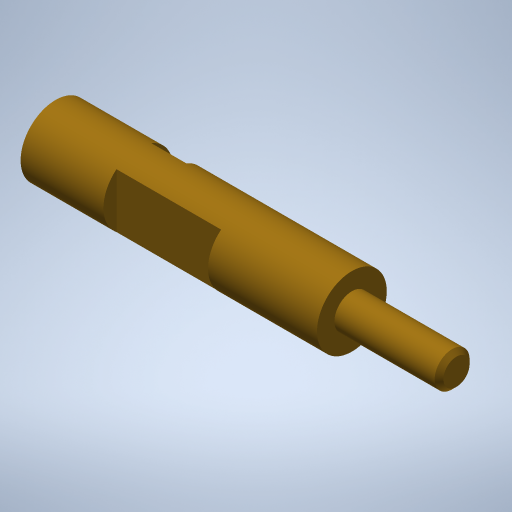
# Autodesk Inventor part: Kurbelwelle
Saved by Autodesk Inventor 2024 (Build 280153000, 153)
## iProperties
Created: 2004-03-27
Part Number: Kurbelwelle
Material: CuZn40
Description: Kurbelwelle
Document SubType Name: Modellieren
Designer: UR
Density: 8.47 g/cm^3
Appearance: Metall - Messing
Control State: 0
Master: False
Checked Out: False
Shininess: 20.0
Angle Display Precision: 2
Document Length Units: 11269
Document Angle Units: 11279
Document Time Units: 11290
Document Mass Units: 11283
Document Length Units Precision: 3
Document Angle Units Precision: 2
Density: 0.0
Volumn: 0.0
Area: 0.0
PropertySet Name: Model Information
Author: UR
Autodesk Inventor part; units mm, degrees
note: some values were not read from the file. Chosen so that the rebuilt part matches the saved one: direction of "3,2 Bohrung radial".
ref_plane "YZ Ebene" through (0, 0, 0) normal (1, 0, 0) x (0, 1, 0)
sketch "Skizze1" plane through (0, 0, 0) normal (0, 0, 1) x (1, 0, 0)
  line L0 (-16.1705, 4.6008) -> (-16.1705, 8.6008)
  line L1 (-16.1705, 8.6008) -> (17.8295, 8.6008)
  line L2 (17.8295, 8.6008) -> (17.8295, 6.6008)
  line L3 (17.8295, 6.6008) -> (29.8295, 6.6008)
  line L4 (29.8295, 6.6008) -> (29.8295, 4.6008)
  line L5 (29.8295, 4.6008) -> (-16.1705, 4.6008)
  dimension "d0" = 46
  dimension "d1" = 12
  dimension "d2" = 4
  dimension "d3" = 8
  constraints: 12 end point, 4 parallel, 1 perpendicular, 1 vertical
  measures "d0" distance of L4.end L0.start
  measures "d1" distance of L2.end L3.end
  measures "d2" diameter of L3 L5
  measures "d3" diameter of L1 L5
revolve "Grundkörper" add sketch "Skizze1" angle 360 about axis through (29.8295, 4.6008, 0) along (-1, 0, 0)
sketch "Skizze2" plane through (-16.1705, 4.6008, 0) normal (-1, 0, 0) x (0, 0, 1)
  circle A0 centre (0, 0) radius 4 projected
  constraints: 1 coincident
hole "3,2 Bohrung axial" at (-16.1705, 4.6008, 0) direction (1, 0, 0) diameter 3.2 depth 14 tip angle 118
chamfer "Fase 0,5x45" distance 0.5 angle 45 1 edges at (29.8295, 2.6008, 0)
ref_plane "Arbeitsebene1" through (0.8295, 8.6008, 0) normal (0, 1, 0) x (-1, 0, 0)
sketch "Skizze3" plane through (0.8295, 8.6008, 0) normal (0, 1, 0) x (-1, 0, 0)
  line L0 (17, 4) -> (17, -4) projected
  point P0 (5.5, 0)
  dimension "d14" = 11.5
  measures "d14" distance from line of L0 point (5.5, 0)
hole "3,2 Bohrung radial" at (-4.6705, 8.6008, 0) direction (0, -1, 0) diameter 3.2 end up to surface
ref_plane "Arbeitsebene2" through (-6.6705, 4.6008, 0) normal (-1, 0, 0) x (0, 0, 1)
sketch "Skizze5" plane through (-6.6705, 4.6008, 0) normal (-1, 0, 0) x (0, 0, 1)
  line L0 (-1.6, 0) -> (-1.6, 3.6661) projected
  circle A0 centre (0, 0) radius 4 projected
  line L1 (1.6, 0) -> (1.6, 3.6661) projected
  line L2 (-3.9383, 0.7) -> (-2.1, 2.5)
  line L3 (-2.1, 2.5) -> (2.1, 2.5)
  line L4 (2.1, 2.5) -> (3.7081, 1.5)
  line L5 (3.1225, -2.5) -> (-3.1225, -2.5)
  line L6 (0, -4) -> (0, 4) construction
  dimension "d31" = 1.5
  dimension "d32" = 4
  dimension "d33" = 3.2
  dimension "d34" = 5
  dimension "d35" = 0.5
  dimension "d36" = 0.5
  constraints: 10 end point, 2 perpendicular, 1 parallel, 7 other
  measures "d31" distance from line of L5 L6.start
  measures "d32" distance from line of L4.end L5
  measures "d33" distance from line of L5 L2.start
  measures "d34" distance between parallel lines of L5 L3
  measures "d35" distance from line of L0 L2.end
  measures "d36" distance from line of L3.end L1
extrude "Entlüftungssteuerschlitz" cut sketch "Skizze5" against normal blind 4 contours L3 L2 A0 L0 | L0 A0 L1 L3 | L1 A0 L4 L3
extrude "Belüftungssteuerschlitz" cut sketch "Skizze5" against normal blind 12 contours L5 A0
